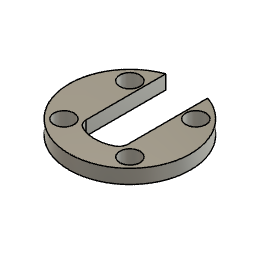
cryo clamp lower v4 (Autodesk Fusion 360 design; units mm, degrees)
Autodesk Fusion 360 part; units mm, degrees
note: some values were not read from the file. Set by a fixed rule: which sketch regions a step uses; the direction of a hole.
sketch "Sketch1" plane through (0, 0, 0) normal (0, 1, 0) x (1, 0, 0)
  circle A0 centre (0, 0) radius 13
  circle A1 centre (0, 0) radius 7.5
  line L0 (-4.5, 12.1963) -> (-4.5, -6)
  line L1 (4.5, -6) -> (4.5, 12.1963)
  circle A2 centre (0, 0) radius 10 construction
  line L2 (0, 0) -> (7.0711, -7.0711)
  line L3 (0, 0) -> (13, 0) construction
  point P0 (7.0711, -7.0711)
  dimension "d1" = 26
  dimension "d2" = 15
  dimension "d3" = 9
  dimension "d4" = 20
  dimension "d12" = 45
  constraint coincident A0.centre A1.centre
  constraint coincident A0 L0.start
  constraint coincident A1 L0.end
  constraint vertical L0
  constraint coincident A1 L1.start
  constraint coincident A0 L1.end
  constraint parallel L0 L1
  constraint horizontal L0.end L1.start
  constraint concentric A1 A2
  constraint coincident A2 P0
  constraint coincident P0 L2.end
  constraint coincident A0 L3.end
  constraint perpendicular L1 L3
  measures "d1" diameter of A0
  measures "d2" diameter of A1
  measures "d3" distance of L0 L1
  measures "d4" diameter of A2
  measures "d12" angle of L2 L3
extrude "Extrude1" add sketch "Sketch1" along normal blind 3 contours A0 A1 L0 L1 | A1 L1 L2 | A1 L0 | A1 L1 L2 picked at (8.8444, -6.7794)
hole "Hole1" at (7.0711, 0, 7.0711) direction (0, 1, 0) diameter 4.3 end through all
pattern_circular "C-Pattern1" count 4 over 360 about axis through (0, 1.75, 0) along (0, 1, 0) of "Hole1"
fillet "Fillet1" radius 2 2 edges at (-4.5, 1.5, 6) (4.5, 1.5, 6)
sketch "Sketch2" plane through (0, 3, 0) normal (0, 1, 0) x (-1, 0, 0)
  circle A0 centre (7.0711, 7.0711) radius 2.15
  circle A1 centre (7.0711, -7.0711) radius 2.15
  circle A2 centre (-7.0711, -7.0711) radius 2.15
  circle A3 centre (-7.0711, 7.0711) radius 2.15
  arc A4 (4.5, -12.1963) -> (-4.5, -12.1963) centre (0, 0) ccw
  line L0 (-4.5, -12.1963) -> (-4.5, 4.899)
  arc A5 (-3.4091, 6.6804) -> (-4.5, 4.899) centre (-2.5, 4.899) ccw
  arc A6 (3.4091, 6.6804) -> (-3.4091, 6.6804) centre (0, 0) ccw
  arc A7 (4.5, 4.899) -> (3.4091, 6.6804) centre (2.5, 4.899) ccw
  line L1 (4.5, 4.899) -> (4.5, -12.1963)
